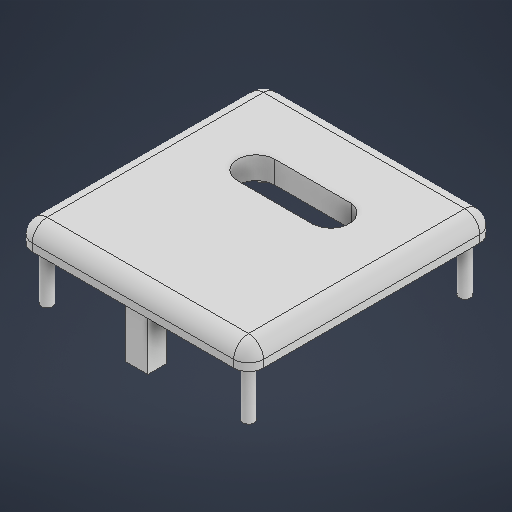
# Autodesk Inventor part: TapaCajaNodoReceptor
Saved by Autodesk Inventor 2027.1 (Build 311270010, 270A)
## iProperties
Created: 2026-09-09
Part Number: TapaCajaNodoReceptor
Material: Genérico
Document SubType Name: Modeling
Designer: marco
Density: 1 g/cm^3
Appearance: Valor por defecto
Author: marco
Autodesk Inventor part; units mm, degrees
ref_plane "YZ Plane" through (0, 0, 0) normal (1, 0, 0) x (0, 1, 0)
ref_plane "XZ Plane" through (0, 0, 0) normal (0, 1, 0) x (-1, 0, 0)
ref_plane "XY Plane" through (0, 0, 0) normal (0, 0, 1) x (1, 0, 0)
sketch "Boceto1" plane through (0, 0, 0) normal (0, 1, 0) x (-1, 0, 0)
  line L0 (15.5, 16.5) -> (-15.5, 16.5)
  line L1 (-15.5, 16.5) -> (-15.5, -16.5)
  line L2 (-15.5, -16.5) -> (15.5, -16.5)
  line L3 (15.5, -16.5) -> (15.5, 16.5)
  line L4 (-15.5, 16.5) -> (15.5, -16.5) construction
  circle A0 centre (15.5, -16.5) radius 0
  line L5 (0, -20.441182) -> (0, -13.180985)
  circle A1 centre (-15.5, -16.5) radius 0
  line L6 (0, 0) -> (-6.703667, 0)
  circle A2 centre (15.5, 16.5) radius 0
  circle A3 centre (-15.5, 16.5) radius 0
  line L7 (-1.743284, -16.5) -> (-1.743284, -13.5)
  line L8 (-1.743284, -13.5) -> (-1.743284, 1.5)
  line L9 (-1.743284, 1.5) -> (-1.743284, 3.5)
  line L10 (-1.743284, 3.5) -> (-1.743284, 13.5)
  line L11 (-1.743284, 13.5) -> (-1.743284, 16.5)
  line L12 (15.5, 0) -> (12.5, 0)
  line L13 (12.5, 0) -> (-12.5, 0)
  line L14 (-12.5, 0) -> (-15.5, 0)
  line L15 (-0.653653, 1.5) -> (-0.653653, -3.5)
  line L16 (12.5, 0) -> (12.5, -5)
  line L17 (12.5, -5) -> (2.466636, -5)
  line L18 (-15.5, 0) -> (-15.5, -5)
  line L19 (-15.5, -5) -> (-12.5, -5)
  circle A4 centre (4.966636, -5) radius 2.5
  line L20 (0, -8.467064) -> (0, -3.5)
  line L21 (12.5, -5) -> (7.5, -5)
  line L22 (12.5, -5) -> (-15.5, -5)
  line L23 (-12.5, -5) -> (-7.5, -5)
  line L24 (-7.5, -5.492671) -> (-7.5, -4.332105)
  line L25 (-7.5, -7.321441) -> (-7.5, -3.5)
  line L26 (-7.5, -5) -> (-3.010459, -5)
  line L27 (-5.25523, -5) -> (-5.25523, -7.5)
  line L28 (-5.25523, -7.5) -> (-3.485236, -7.5)
  line L29 (-5.25523, -5) -> (-5.25523, -2.5)
  line L30 (-5.25523, -2.5) -> (-3.924845, -2.5)
  circle A5 centre (-5, -5) radius 2.5
  line L31 (4.966636, -7.5) -> (-5.25523, -7.5)
  line L32 (-5.25523, -2.5) -> (4.966636, -2.5)
  point P0 (-5.25523, -2.513063)
  point P1 (-5.25523, -7.486937)
  dimension "d0" = 31
  dimension "d1" = 33
  dimension "d3" = 3
  dimension "d4" = 15
  dimension "d5" = 2
  dimension "d6" = 10
  dimension "d7" = 3
  dimension "d8" = 3
  dimension "d9" = 25
  dimension "d10" = 3
  dimension "d11" = 5
  dimension "d12" = 5
  dimension "d14" = 5
  dimension "d15" = 3
  dimension "d16" = 5
  dimension "d17" = 5
  dimension "d19" = 5
  dimension "d21" = 2.5
  dimension "d22" = 2.5
  constraints: 66 end point, 11 point on line, 7 vertical, 6 centre point, 6 tangent, 5 perpendicular, 4 horizontal, 4 midpoint, 3 parallel, 3 point on circle, 3 symmetric about line, 1 collinear, 3 other
  measures "d0" distance of L2.end L1.end
  measures "d1" distance of L1.end L0.end
  measures "d3" distance of L7.start L7.end
  measures "d4" distance of L7.end L8.end
  measures "d5" distance of L8.end L9.end
  measures "d6" distance of L9.end L10.end
  measures "d7" distance of L10.end L11.end
  measures "d8" distance of L12.start L12.end
  measures "d9" distance of L12.end L13.end
  measures "d10" distance of L13.end L14.end
  measures "d11" distance of L15.start L15.end
  measures "d12" distance of L12.end L16.end
  measures "d14" distance of L14.end L18.end
  measures "d15" distance of L18.end L19.end
  measures "d16" diameter of A4
  measures "d17" distance of L16.end L21.end
  measures "d19" distance of L19.end L23.end
  measures "d21" distance of L27.start L27.end
  measures "d22" distance of L27.start L29.end
sketch "Boceto1 outline for Extrusión1" plane through (0, 0, 0) normal (0, 1, 0) x (-1, 0, 0)
  line L0 (-15.5, -16.5) -> (15.5, -16.5)
  line L1 (-15.5, 16.5) -> (-15.5, -16.5)
  line L2 (15.5, -16.5) -> (15.5, 16.5)
  line L3 (15.5, 16.5) -> (-15.5, 16.5)
  arc A0 (-5.25523, -7.486937) -> (-5.25523, -2.513063) centre (-5, -5) cw
  line L4 (-5.25523, -7.5) -> (-5.25523, -7.486937)
  line L5 (-3.485236, -7.5) -> (-5.25523, -7.5)
  line L6 (4.966636, -7.5) -> (-3.485236, -7.5)
  arc A1 (4.966636, -2.5) -> (4.966636, -7.5) centre (4.966636, -5) cw
  line L7 (-3.924845, -2.5) -> (4.966636, -2.5)
  line L8 (-5.25523, -2.5) -> (-3.924845, -2.5)
  line L9 (-5.25523, -2.513063) -> (-5.25523, -2.5)
extrude "Extrusión1" add sketch "Boceto1 outline for Extrusión1" along normal blind 3
fillet "Empalme1" radius 2 8 edges at (-15.5, 1.5, 16.5) (-15.5, 3, 0) (-15.5, 1.5, -16.5) (0, 3, -16.5) (15.5, 3, 0) (0, 3, 16.5) (15.5, 1.5, 16.5) (15.5, 1.5, -16.5)
sketch "Boceto2" plane through (0, 0, 0) normal (0, -1, 0) x (1, 0, 0)
  line L0 (-13.5, -14.5) -> (13.5, -14.5)
  circle A0 centre (13.5, -14.5) radius 0.75
  line L1 (0, -0.514663) -> (0, 1.763645)
  circle A1 centre (-13.5, -14.5) radius 0.75
  line L2 (0.998187, 0) -> (-3.186461, 0)
  circle A2 centre (13.5, 14.5) radius 0.75
  circle A3 centre (-13.5, 14.5) radius 0.75
  arc A4 (15.5, 14.5) -> (13.5, 16.5) centre (13.5, 14.5) ccw
  arc A5 (-13.5, 16.5) -> (-15.5, 14.5) centre (-13.5, 14.5) ccw
  arc A6 (-15.5, -14.5) -> (-13.5, -16.5) centre (-13.5, -14.5) ccw
  arc A7 (13.5, -16.5) -> (15.5, -14.5) centre (13.5, -14.5) ccw
  line L3 (-15.5, -14.5) -> (-15.5, 14.5)
  line L4 (-15.5, -14.5) -> (-1.5, -14.5)
  line L5 (-1.5, -14.5) -> (1, -14.5)
  line L6 (13.5, -14.5) -> (13.5, -13.5)
  line L7 (13.5, -14.5) -> (13.5, 14.5)
  line L8 (13.5, -13.5) -> (-13.5, -13.5)
  line L9 (-13.5, 14.5) -> (-13.5, -14.5)
  line L10 (15.5, 14.5) -> (15.5, -14.5)
  line L11 (15.5, -13.5) -> (1.5, -13.5)
  line L12 (-15.5, -13.5) -> (-1.5, -13.5)
  line L13 (1.5, -13.5) -> (1.5, -16)
  line L14 (1.5, -16) -> (-1.5, -16)
  line L15 (-1.5, -16) -> (-1.5, -13.5)
  line L16 (-1.5, 14.5) -> (1, 14.5)
  line L17 (1.5, 13.5) -> (1.5, 16)
  line L18 (1.5, 16) -> (-1.5, 16)
  line L19 (-1.5, 16) -> (-1.5, 13.5)
  line L20 (13.5, 14.5) -> (-13.5, 14.5)
  line L21 (0.770935, 14.5) -> (1.5, 14.5)
  line L22 (-1.5, 16) -> (-1.5, 13.5)
  line L23 (1.5, 13.5) -> (-1.5, 13.5)
  dimension "d26" = 1.5
  dimension "d27" = 14
  dimension "d28" = 2.5
  dimension "d29" = 1
  dimension "d30" = 14
  dimension "d31" = 14
  dimension "d32" = 2.5
  constraints: 36 end point, 11 point on line, 8 symmetric about line, 4 centre point, 4 concentric, 3 perpendicular, 2 vertical, 1 collinear, 1 horizontal, 1 parallel, 3 other
  measures "d26" diameter of A0
  measures "d27" distance of L3.start L4.end
  measures "d28" distance of L4.end L5.end
  measures "d29" distance of L6.start L6.end
  measures "d30" distance of L11.start L11.end
  measures "d31" distance of L12.start L12.end
  measures "d32" distance of L11.end L13.end
extrude "Extrusión2" add sketch "Boceto2" along normal blind 7 contours L9 A1 L0 | L0 A1 L4 | L4 A1 L9 | L15 L8 L13 L0 | L0 L13 L14 L15 | L9 L20 A3 | A3 L20 L9 | A0 L6 L0 | L0 L6 A0 | L19 L18 L17 L20 L16 | L16 L20 L17 L23 L19 | L7 L20 A2 | A2 L20 L7
